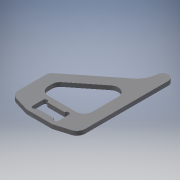
# Autodesk Inventor part: 上腕_サブフレーム_1_1
Saved by Autodesk Inventor 2018 (Build 220112000, 112)
## iProperties
Created: 2016-05-04
Part Number: 上腕_サブフレーム_1_1
Material: GFRP
Document SubType Name: Modeling
Designer: hiroaki
Density: 1.75 g/cm^3
Appearance: 滑らか - 淡い灰色
Mass: 2.29994 g
Surface Area: 19.0417 cm^2
Volume: 1.31425 cm^3
Author: hiroaki
Autodesk Inventor part; units mm, degrees
ref_plane "YZ Plane" through (0, 0, 0) normal (1, 0, 0) x (0, 1, 0)
ref_plane "XZ Plane" through (0, 0, 0) normal (0, 1, 0) x (-1, 0, 0)
ref_plane "XY Plane" through (0, 0, 0) normal (0, 0, 1) x (1, 0, 0)
sketch "スケッチ1" plane through (0, 0, 0) normal (0, 0, 1) x (1, 0, 0)
  line L0 (-13.5, 13.5) -> (13.5, 13.5) construction
  line L1 (13.5, 13.5) -> (13.5, -13.5) construction
  line L2 (13.5, -13.5) -> (-13.5, -13.5) construction
  line L3 (-13.5, -13.5) -> (-13.5, 13.5) construction
  circle A0 centre (-13.5, 13.5) radius 1.35
  circle A1 centre (13.5, 13.5) radius 1.35
  circle A2 centre (-13.5, -13.5) radius 1.35
  circle A3 centre (13.5, -13.5) radius 1.35
  circle A4 centre (0, 14.5) radius 10.5 construction
  line L4 (-6.25, -25) -> (6.25, -25) construction
  line L5 (6.25, -25) -> (6.25, -30) construction
  line L6 (6.25, -30) -> (-6.25, -30) construction
  line L7 (-6.25, -30) -> (-6.25, -25) construction
  line L8 (-16.25, -25) -> (16.25, -25) construction
  line L9 (16.25, -25) -> (16.25, -30) construction
  line L10 (16.25, -30) -> (-16.25, -30) construction
  line L11 (-16.25, -30) -> (-16.25, -25) construction
  line L12 (-6.3, -24.95) -> (6.3, -24.95) construction
  line L13 (6.3, -24.95) -> (6.3, -30.05) construction
  line L14 (6.3, -30.05) -> (-6.3, -30.05) construction
  line L15 (-6.3, -30.05) -> (-6.3, -24.95) construction
  circle A5 centre (-5.25, -24.95) radius 1.05 construction
  circle A6 centre (-11.25, -27.5) radius 1.55
  circle A7 centre (11.25, -27.5) radius 1.55
  line L16 (0, 0) -> (0, -13.5) construction
  line L17 (-6.3, -24.95) -> (-6.3, -30.05)
  line L18 (6.3, -27.5) -> (-6.3, -27.5) construction
  line L19 (0, -25) -> (0, -30.05) construction
  arc A8 (-4.2, -24.95) -> (-6.3, -24.95) centre (-5.25, -24.95) ccw
  arc A9 (-6.3, -30.05) -> (-4.2, -30.05) centre (-5.25, -30.05) ccw
  line L20 (-4.2, -24.95) -> (4.2, -24.95)
  line L21 (-4.2, -30.05) -> (4.2, -30.05)
  arc A10 (6.3, -24.95) -> (4.2, -24.95) centre (5.25, -24.95) ccw
  arc A11 (4.2, -30.05) -> (6.3, -30.05) centre (5.25, -30.05) ccw
  line L22 (6.3, -24.95) -> (6.3, -30.05)
  circle A12 centre (-13.5, -13.5) radius 2.75 construction
  circle A13 centre (13.5, 13.5) radius 2.75 construction
  line L23 (-16.25, -13.5) -> (-16.25, -30)
  line L24 (-16.25, -30) -> (-6.25, -33)
  line L25 (-6.25, -33) -> (6.25, -33)
  line L26 (6.25, -33) -> (16.25, -30)
  line L27 (16.25, -30) -> (16.25, 13.5)
  arc A14 (16.25, 13.5) -> (10.7575, 13.7031) centre (13.5, 13.5) ccw
  arc A15 (6.7066, 6.0513) -> (10.7575, 13.7031) centre (0, 14.5) ccw
  line L28 (6.7066, 6.0513) -> (-15.2098, -11.3461)
  arc A16 (-15.2098, -11.3461) -> (-16.25, -13.5) centre (-13.5, -13.5) ccw
  line L29 (-10.75, -14.1897) -> (-10.75, -22)
  line L30 (-10.75, -22) -> (10.75, -22)
  line L31 (10.75, -22) -> (10.75, 2.8772)
  line L32 (10.75, 2.8772) -> (-10.75, -14.1897)
  point P0 (0, 13.5)
  point P1 (13.5, 0)
  point P2 (-16.25, -27.5)
  dimension "d23" = 2.1
  dimension "d0" = 27
  dimension "d3" = 27
  dimension "d6" = 27
  dimension "d9" = 2.7
  dimension "d10" = 21
  dimension "d11" = 1
  dimension "d12" = 11.5
  dimension "d13" = 5
  dimension "d16" = 32.5
  dimension "d20" = 10
  dimension "d22" = 0.05
  dimension "d24" = 5
  dimension "d26" = 3.1
  dimension "d31" = 5.5
  dimension "d32" = 3
  dimension "d33" = 5
  dimension "d34" = 3
  constraints: 66 end point, 16 centre point, 14 point on circle, 12 parallel, 10 tangent, 9 midpoint, 8 coincident, 8 perpendicular, 5 horizontal, 5 symmetric about line, 4 collinear, 4 horizontal alignment, 4 vertical, 4 vertical alignment, 2 concentric, 1 equal radius, 1 point on line, 15 other
  measures "d0" distance of L0.end L1.end
  measures "d3" distance of A0.centre A1.centre
  measures "d6" distance of A0.centre A2.centre
  measures "d9" diameter of A0
  measures "d10" diameter of A4
  measures "d11" distance from line of L0 A4.centre
  measures "d12" distance from line of L1.end L4
  measures "d13" distance of L4.end L5.end
  measures "d16" distance of L10.end L9.end
  measures "d20" distance between parallel lines of L11 L7
  measures "d22" distance between parallel lines of L15 L7
  measures "d24" distance from line of L11 A6.centre
  measures "d26" diameter of A6
  measures "d31" diameter of A13
  measures "d32" distance between parallel lines of L10 L25
  measures "d33" distance between parallel lines of L32 L28
  measures "d34" distance between parallel lines of L30 L8
extrude "押し出し1" add sketch "スケッチ1" along normal blind 2 contours A16 L28 A15 A14 L27 L26 L25 L24 L23
fillet "フィレット1" radius 4 8 edges at (10.75, 2.8772, 1) (-10.75, -22, 1) (-10.75, -14.1897, 1) (10.75, -22, 1) (16.25, -30, 1) (-16.25, -30, 1) (-6.25, -33, 1) (6.25, -33, 1)
sketch "スケッチ2" plane through (0, 0, 2) normal (0, 0, 1) x (1, 0, 0)
  circle A0 centre (-13.5, -13.5) radius 1.35 projected
  circle A1 centre (-13.5, -13.5) radius 1.35
  circle A2 centre (13.5, -13.5) radius 1.35 projected
  circle A3 centre (13.5, -13.5) radius 1.35
  circle A4 centre (11.25, -27.5) radius 1.55 projected
  circle A5 centre (11.25, -27.5) radius 1.55
  circle A6 centre (-11.25, -27.5) radius 1.55 projected
  circle A7 centre (-11.25, -27.5) radius 1.55
  circle A8 centre (13.5, 13.5) radius 1.35 projected
  circle A9 centre (13.5, 13.5) radius 1.35
  point P0 (0, 0)
  constraints: 5 centre point, 5 coincident
extrude "押し出し2" add sketch "スケッチ2" against normal up to surface (2 mm away)
equation "\"d3\" = d0"
equation "\"d6\" = d0"
equation "\"d16\" = d0_1"
equation "\"d20\" = d3_1"
equation "\"d24\" = d17"
equation "\"d34\" = d32"
equation "\"d0_1\" = 32.5"
equation "\"d3_1\" = 10"
equation "\"d17\" = 5"
